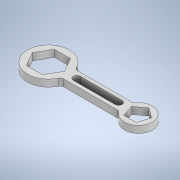
# Autodesk Inventor part: Exercise_2
Saved by Autodesk Inventor 2020 (Build 240168000, 168)
## iProperties
Created: 2022-11-07
Part Number: Exercise_2
Material: Generic
Document SubType Name: Modeling
Designer: Matthew Ng
Density: 1 g/cm^3
Appearance: Default
Author: Matthew Ng
Autodesk Inventor part; units mm, degrees
ref_plane "YZ Plane" through (0, 0, 0) normal (1, 0, 0) x (0, 1, 0)
ref_plane "XZ Plane" through (0, 0, 0) normal (0, 1, 0) x (-1, 0, 0)
ref_plane "XY Plane" through (0, 0, 0) normal (0, 0, 1) x (1, 0, 0)
sketch "Sketch2" plane through (0, 0, 0) normal (0, 1, 0) x (-1, 0, 0)
  arc A0 (-27.1052, -12.8571) -> (-27.1052, 12.8571) centre (0, 0) ccw
  line L0 (-23.094, 0) -> (-11.547, 20)
  line L1 (-11.547, 20) -> (11.547, 20)
  line L2 (11.547, 20) -> (23.094, 0)
  line L3 (23.094, 0) -> (11.547, -20)
  line L4 (11.547, -20) -> (-11.547, -20)
  line L5 (-11.547, -20) -> (-23.094, 0)
  line L6 (-184.8904, 0) -> (65.8151, 0) projected
  arc A1 (-112.9549, 12.0151) -> (-113.0454, -11.9849) centre (-129, 0.0754) ccw
  line L7 (-129, -14.9246) -> (-143.2658, -4.5598)
  line L8 (-143.2658, -4.5598) -> (-137.8168, 12.2107)
  line L9 (-137.8168, 12.2107) -> (-120.1832, 12.2107)
  line L10 (-120.1832, 12.2107) -> (-114.7342, -4.5598)
  line L11 (-114.7342, -4.5598) -> (-129, -14.9246)
  line L12 (-31.6228, -10) -> (-109.0568, -10)
  line L13 (-108.9436, 10) -> (-31.6228, 10)
  line L14 (-40.4814, 0) -> (-100.4814, 0) construction
  line L15 (-40.4814, 5) -> (-100.4814, 5)
  line L16 (-100.4814, -5) -> (-40.4814, -5)
  arc A2 (-40.4814, -5) -> (-40.4814, 5) centre (-40.4814, 0) ccw
  arc A3 (-100.4814, 5) -> (-100.4814, -5) centre (-100.4814, 0) ccw
  arc A4 (-27.1052, -12.8571) -> (-31.6228, -10) centre (-31.6228, -15) ccw
  arc A5 (-31.6228, 10) -> (-27.1052, 12.8571) centre (-31.6228, 15) ccw
  arc A6 (-109.0568, -10) -> (-113.0454, -11.9849) centre (-109.0568, -15) ccw
  arc A7 (-112.9549, 12.0151) -> (-108.9436, 10) centre (-108.9436, 15) ccw
  point P0 (-28.2843, -10)
  point P1 (-111.6362, 10)
  point P2 (-111.7233, -10)
  point P3 (-70.4814, 0)
  point P4 (-28.2843, 10)
  dimension "d14" = 60
  dimension "d15" = 20
  dimension "d16" = 40
  dimension "d17" = 15
  dimension "d24" = 129
  dimension "d25" = 60
  dimension "d26" = 10
  dimension "d27" = 5
  dimension "d28" = 5
  constraints: 34 end point, 20 point on circle, 12 tangent, 8 centre point, 6 point on line, 3 coincident, 2 equal radius, 2 parallel, 1 horizontal, 1 midpoint, 24 other
  measures "d14" diameter of A0
  measures "d15" distance between parallel lines of L6 L4
  measures "d16" diameter of A1
  measures "d17" distance of point (-129, 0.075) L7.start
  measures "d24" distance of A1.centre A0.centre
  measures "d25" distance of L14.start L14.end
  measures "d26" diameter of A3
  measures "d27" radius of A4
  measures "d28" radius of A5
extrude "Extrusion1" add sketch "Sketch2" along normal blind 10 contours A4 L12 A6 A1 L6 L8 L7 L11 L10 A3 L16 A2 L5 L4 L3 A0 | L6 L2 L1 L0 A2 L15 A3 L10 L9 L8 A1 A7 L13 A5 A0
body "Solid1"
